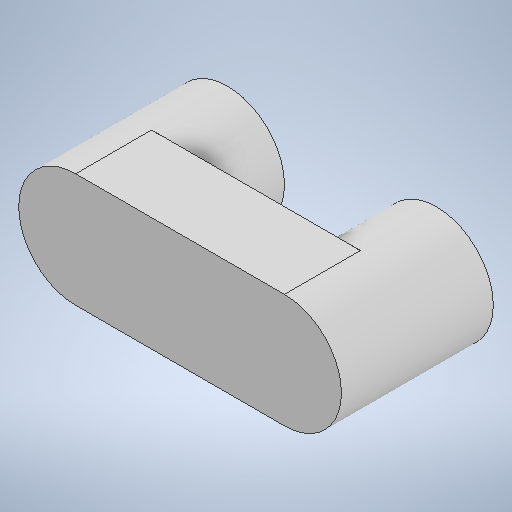
# Autodesk Inventor part: ModuleConnector_Axis_Connector
Saved by Autodesk Inventor 2025.1 (Build 291241020, 241B)
## iProperties
Created: 2024-10-09
Part Number: ModuleConnector_Axis_Connector
Material: 일반
Document SubType Name: Modeling
Designer: SEON06
Density: 1 g/cm^3
Appearance: 기본값
Author: SEON06
Autodesk Inventor part; units mm, degrees
ref_plane "YZ Plane" through (0, 0, 0) normal (1, 0, 0) x (0, 1, 0)
ref_plane "XZ Plane" through (0, 0, 0) normal (0, 1, 0) x (-1, 0, 0)
ref_plane "XY Plane" through (0, 0, 0) normal (0, 0, 1) x (1, 0, 0)
sketch "스케치1" plane through (0, 0, 0) normal (0, 0, 1) x (1, 0, 0)
  circle A0 centre (0, 0) radius 1.5
  circle A1 centre (5.5, 0) radius 1.5
  line L0 (0, 1.5) -> (5.5, 1.5)
  line L1 (0, -1.5) -> (5.5, -1.5)
  dimension "d0" = 5.5
  dimension "d1" = 3
  constraints: 4 end point, 4 point on circle, 2 centre point, 2 horizontal, 2 tangent, 1 coincident, 1 equal radius, 1 horizontal alignment
  measures "d0" distance of A1.centre point (0, 0)
  measures "d1" diameter of A1
extrude "돌출1" add sketch "스케치1" along normal blind 2
extrude "돌출2" add sketch "스케치1" against normal blind 2 contours A0 | A1
